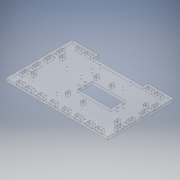
# Autodesk Inventor part: case_base
Saved by Autodesk Inventor 2019 (Build 230136000, 136)
## iProperties
Created: 2019-02-02
Part Number: case_base
Material: Acrylic, Clear
Document SubType Name: Modeling
Designer: suchanek
Density: 1.19 g/cm^3
Appearance: Transparent - Clear
Author: suchanek
Autodesk Inventor part; units mm, degrees
ref_plane "YZ Plane" through (0, 0, 0) normal (1, 0, 0) x (0, 1, 0)
ref_plane "XZ Plane" through (0, 0, 0) normal (0, 1, 0) x (-1, 0, 0)
ref_plane "XY Plane" through (0, 0, 0) normal (0, 0, 1) x (1, 0, 0)
sketch "Sketch1" plane through (0, 0, 0) normal (0, 1, 0) x (-1, 0, 0)
  line L0 (100, 65) -> (-100, 65)
  line L1 (-100, 65) -> (-100, -65)
  line L2 (-100, -65) -> (100, -65)
  line L3 (100, -65) -> (100, 65)
  line L4 (100, 65) -> (-100, -65) construction
  line L5 (-100, 65) -> (100, -65) construction
  line L6 (0, 0) -> (4.5236, 0)
  line L7 (0, 8) -> (0, -18)
  circle A0 centre (58.5, -13.1) radius 1
  circle A1 centre (30.6, -13.1) radius 1
  circle A2 centre (73.7, 37.7) radius 1
  circle A3 centre (25.5, 39) radius 1
  circle A4 centre (15, 28) radius 2.6
  circle A5 centre (15, -28) radius 2.6
  line L8 (0, 0) -> (5.2635, 0)
  circle A6 centre (-15, 28) radius 2.6
  circle A7 centre (-15, -28) radius 2.6
  line L9 (48.5, 0) -> (48.5, 7.3763)
  line L10 (-48.5, 0) -> (-48.5, 7.3763)
  circle A8 centre (-82, 28) radius 2.6
  circle A9 centre (-82, -28) radius 2.6
  circle A10 centre (82, 28) radius 2.6
  circle A11 centre (82, -28) radius 2.6
  line L11 (96, -42) -> (90, -42)
  line L12 (90, -42) -> (90, -30)
  line L13 (90, -30) -> (96, -30)
  line L14 (96, -30) -> (96, -42)
  line L15 (96, -18) -> (90, -18)
  line L16 (90, -18) -> (90, -6)
  line L17 (90, -6) -> (96, -6)
  line L18 (96, -6) -> (96, -18)
  line L19 (66, -55) -> (54, -55)
  line L20 (54, -55) -> (54, -61)
  line L21 (54, -61) -> (66, -61)
  line L22 (66, -61) -> (66, -55)
  line L23 (72, -61) -> (84, -61)
  line L24 (84, -61) -> (84, -55)
  line L25 (84, -55) -> (72, -55)
  line L26 (72, -55) -> (72, -61)
  line L27 (-96, -42) -> (-90, -42)
  line L28 (-90, -42) -> (-90, -30)
  line L29 (-90, -30) -> (-96, -30)
  line L30 (-96, -30) -> (-96, -42)
  line L31 (-96, -18) -> (-90, -18)
  line L32 (-90, -18) -> (-90, -6)
  line L33 (-90, -6) -> (-96, -6)
  line L34 (-96, -6) -> (-96, -18)
  line L35 (-66, -55) -> (-54, -55)
  line L36 (-54, -55) -> (-54, -61)
  line L37 (-54, -61) -> (-66, -61)
  line L38 (-66, -61) -> (-66, -55)
  line L39 (-72, -61) -> (-84, -61)
  line L40 (-84, -61) -> (-84, -55)
  line L41 (-84, -55) -> (-72, -55)
  line L42 (-72, -55) -> (-72, -61)
  line L43 (96, 42) -> (90, 42)
  line L44 (90, 42) -> (90, 30)
  line L45 (90, 30) -> (96, 30)
  line L46 (96, 30) -> (96, 42)
  line L47 (96, 18) -> (90, 18)
  line L48 (90, 18) -> (90, 6)
  line L49 (90, 6) -> (96, 6)
  line L50 (96, 6) -> (96, 18)
  line L51 (66, 55) -> (54, 55)
  line L52 (54, 55) -> (54, 61)
  line L53 (54, 61) -> (66, 61)
  line L54 (66, 61) -> (66, 55)
  line L55 (42, 55) -> (30, 55)
  line L56 (30, 55) -> (30, 61)
  line L57 (30, 61) -> (42, 61)
  line L58 (42, 61) -> (42, 55)
  line L59 (18, 55) -> (6, 55)
  line L60 (6, 55) -> (6, 61)
  line L61 (6, 61) -> (18, 61)
  line L62 (18, 61) -> (18, 55)
  line L63 (72, 61) -> (84, 61)
  line L64 (84, 61) -> (84, 55)
  line L65 (84, 55) -> (72, 55)
  line L66 (72, 55) -> (72, 61)
  line L67 (-90, 30) -> (-96, 30)
  line L68 (-96, 18) -> (-90, 18)
  line L69 (-90, 18) -> (-90, 6)
  line L70 (-90, 6) -> (-96, 6)
  line L71 (-96, 6) -> (-96, 18)
  line L72 (-96, 42) -> (-90, 42)
  line L73 (-96, 30) -> (-96, 42)
  line L74 (-90, 42) -> (-90, 30)
  line L75 (-84, 55) -> (-72, 55)
  line L76 (-84, 61) -> (-84, 55)
  line L77 (-72, 61) -> (-84, 61)
  line L78 (-72, 55) -> (-72, 61)
  line L79 (-66, 61) -> (-66, 55)
  line L80 (-54, 55) -> (-54, 61)
  line L81 (-54, 61) -> (-66, 61)
  line L82 (-66, 55) -> (-54, 55)
  line L83 (-6, 55) -> (-6, 61)
  line L84 (-18, 55) -> (-6, 55)
  line L85 (-6, 61) -> (-18, 61)
  line L86 (-18, 61) -> (-18, 55)
  line L87 (-30, 55) -> (-30, 61)
  line L88 (-42, 61) -> (-42, 55)
  line L89 (-30, 61) -> (-42, 61)
  line L90 (-42, 55) -> (-30, 55)
  line L91 (82, 25.5) -> (82, 30.5) construction
  line L92 (84.6, 25.5) -> (84.6, 30.5)
  line L93 (79.4, 30.5) -> (79.4, 25.5)
  arc A12 (79.4, 25.5) -> (84.6, 25.5) centre (82, 25.5) ccw
  arc A13 (84.6, 30.5) -> (79.4, 30.5) centre (82, 30.5) ccw
  line L94 (12.4, 25.5) -> (12.4, 30.5)
  line L95 (17.6, 30.5) -> (17.6, 25.5)
  arc A14 (12.4, 25.5) -> (17.6, 25.5) centre (15, 25.5) ccw
  arc A15 (17.6, 30.5) -> (12.4, 30.5) centre (15, 30.5) ccw
  line L96 (-84.6, 25.5) -> (-84.6, 30.5)
  line L97 (-79.4, 30.5) -> (-79.4, 25.5)
  arc A16 (-84.6, 25.5) -> (-79.4, 25.5) centre (-82, 25.5) ccw
  arc A17 (-79.4, 30.5) -> (-84.6, 30.5) centre (-82, 30.5) ccw
  arc A18 (-17.6, 25.5) -> (-12.4, 25.5) centre (-15, 25.5) ccw
  line L98 (-12.4, 25.5) -> (-12.4, 30.5)
  line L99 (-17.6, 30.5) -> (-17.6, 25.5)
  arc A19 (-12.4, 30.5) -> (-17.6, 30.5) centre (-15, 30.5) ccw
  line L100 (82, -25.5) -> (82, -30.5) construction
  line L101 (84.6, -25.5) -> (84.6, -30.5)
  line L102 (79.4, -30.5) -> (79.4, -25.5)
  arc A20 (84.6, -25.5) -> (79.4, -25.5) centre (82, -25.5) ccw
  arc A21 (79.4, -30.5) -> (84.6, -30.5) centre (82, -30.5) ccw
  arc A22 (17.6, -25.5) -> (12.4, -25.5) centre (15, -25.5) ccw
  line L103 (12.4, -25.5) -> (12.4, -30.5)
  line L104 (17.6, -30.5) -> (17.6, -25.5)
  arc A23 (12.4, -30.5) -> (17.6, -30.5) centre (15, -30.5) ccw
  line L105 (-84.6, -25.5) -> (-84.6, -30.5)
  arc A24 (-84.6, -30.5) -> (-79.4, -30.5) centre (-82, -30.5) ccw
  line L106 (-79.4, -30.5) -> (-79.4, -25.5)
  arc A25 (-79.4, -25.5) -> (-84.6, -25.5) centre (-82, -25.5) ccw
  arc A26 (-12.4, -25.5) -> (-17.6, -25.5) centre (-15, -25.5) ccw
  line L107 (-17.6, -30.5) -> (-17.6, -25.5)
  line L108 (-12.4, -25.5) -> (-12.4, -30.5)
  arc A27 (-17.6, -30.5) -> (-12.4, -30.5) centre (-15, -30.5) ccw
  line L109 (-55, 14) -> (10, 14)
  line L110 (10, 14) -> (10, -14)
  line L111 (10, -14) -> (-55, -14)
  line L112 (-55, -14) -> (-55, 14)
  circle A28 centre (-60, -6) radius 2.15
  circle A29 centre (-60, 6) radius 2.15
  line L113 (48, -65) -> (-48, -65)
  line L114 (-48, -65) -> (-48, -55)
  line L115 (-48, -55) -> (48, -55)
  line L116 (48, -55) -> (48, -65)
  line L117 (-22.5, 6) -> (-22.5, -5)
  circle A30 centre (15, -6) radius 2.15
  circle A31 centre (15, 6) radius 2.15
  circle A32 centre (30, -50) radius 1
  circle A33 centre (30, -35) radius 1
  circle A34 centre (-30, -35) radius 1
  circle A35 centre (-30, -50) radius 1
  circle A36 centre (93, -24) radius 1.5
  circle A37 centre (93, 24) radius 1.5
  circle A38 centre (-93, -24) radius 1.5
  circle A39 centre (-93, 24) radius 1.5
  circle A40 centre (48, 58) radius 1.5
  circle A41 centre (-48, 58) radius 1.5
  point P0 (0, 0)
  point P1 (0, 0)
  point P2 (15, -28)
  point P3 (-15, -28)
  point P4 (-82, -28)
  point P5 (82, -28)
  dimension "d0" = 130
  dimension "d1" = 200
  dimension "d7" = 2
  dimension "d8" = 5.1
  dimension "d9" = 27.9
  dimension "d10" = 1.3
  dimension "d11" = 50.8
  dimension "d12" = 15.2
  dimension "d14" = 26
  dimension "d22" = 56
  dimension "d23" = 5.2
  dimension "d31" = 6
  dimension "d32" = 4
  dimension "d34" = 6
  dimension "d35" = 12
  dimension "d36" = 12
  dimension "d37" = 12
  dimension "d43" = 12
  dimension "d44" = 6
  dimension "d45" = 12
  dimension "d50" = 2.5
  dimension "d54" = 10.5
  dimension "d55" = 28
  dimension "d56" = 65
  dimension "d58" = 5
  dimension "d61" = 6
  dimension "d62" = 12
  dimension "d63" = 4.3
  dimension "d64" = 12
  dimension "d65" = 12
  dimension "d66" = 6
  dimension "d67" = 12
  dimension "d68" = 12
  dimension "d69" = 12
  dimension "d70" = 12
  dimension "d71" = 12
  dimension "d72" = 12
  dimension "d73" = 4
  dimension "d74" = 6
  dimension "d75" = 6
  dimension "d76" = 10
  dimension "d77" = 15
  dimension "d78" = 67
  dimension "d79" = 5
  dimension "d80" = 15
  dimension "d81" = 60
  dimension "d82" = 3
  dimension "d83" = 6
  dimension "d84" = 3
  dimension "d85" = 3
  dimension "d86" = 3
  dimension "d87" = 3
  dimension "d88" = 6
  constraints: 240 end point, 108 symmetric about line, 42 centre point, 32 point on circle, 16 parallel, 14 point on line, 10 collinear, 9 equal radius, 9 horizontal, 8 vertical, 7 midpoint, 7 perpendicular, 5 tangent, 4 horizontal alignment, 3 vertical alignment, 28 other
  measures "d0" distance of L2.end L0.start
  measures "d1" distance of L1.end L2.end
  measures "d7" diameter of A1
  measures "d8" horizontal distance of A3.centre A1.centre
  measures "d9" distance of A1.centre A0.centre
  measures "d10" vertical distance of A2.centre A3.centre
  measures "d11" vertical distance of A0.centre A2.centre
  measures "d12" horizontal distance of A2.centre A0.centre
  measures "d14" distance from line of L0 A3.centre
  measures "d22" distance of A5.centre A4.centre
  measures "d23" diameter of A4
  measures "d31" distance between parallel lines of L16 L18
  measures "d32" distance between parallel lines of L3 L18
  measures "d34" distance between parallel lines of L17 L8
  measures "d35" distance of L17.end L15.start
  measures "d36" distance between parallel lines of L15 L13
  measures "d37" distance of L13.end L11.start
  measures "d43" distance of L19.start L19.end
  measures "d44" distance between parallel lines of L22 L26
  measures "d45" distance of L24.end L25.end
  measures "d50" distance of A10.centre L91.end
  measures "d54" horizontal distance of A4.centre A3.centre
  measures "d55" distance of L109.end L110.end
  measures "d56" distance of L110.end L111.end
  measures "d58" distance from line of L112 A29.centre
  measures "d61" distance from line of L6 A29.centre
  measures "d62" distance of A28.centre A29.centre
  measures "d63" diameter of A29
  measures "d64" distance between parallel lines of L58 L52
  measures "d65" distance of L56.end L58.start
  measures "d66" distance of L56.start L56.end
  measures "d67" distance between parallel lines of L62 L56
  measures "d68" distance of L61.start L62.start
  measures "d69" distance between parallel lines of L83 L60
  measures "d70" distance of L83.end L85.end
  measures "d71" distance between parallel lines of L87 L86
  measures "d72" distance of L87.end L89.end
  measures "d73" distance between parallel lines of L0 L61
  measures "d74" distance between parallel lines of L116 L20
  measures "d75" distance between parallel lines of L36 L114
  measures "d76" distance between parallel lines of L110 L7
  measures "d77" distance from line of L7 A4.centre
  measures "d78" distance of A8.centre A6.centre
  measures "d79" distance from line of L115 A32.centre
  measures "d80" distance of A32.centre A33.centre
  measures "d81" distance of A35.centre A32.centre
  measures "d82" diameter of A36
  measures "d83" distance from line of L13 A36.centre
  measures "d84" distance from line of L14 A36.centre
  measures "d85" diameter of A40
  measures "d86" diameter of A41
  measures "d87" distance from line of L53 A40.centre
  measures "d88" distance from line of L58 A40.centre
extrude "Extrusion3" add sketch "Sketch1" along normal blind 6 contours L3 L2 L116 L115 L114 L1 L0
body "Solid3"
